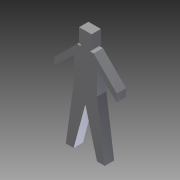
# Autodesk Inventor part: Human_5ft_9in
Saved by Autodesk Inventor 2012 (Build 160160000, 160)
## iProperties
Created: 2013-07-14
Part Number: Human_5ft_9in
Material: Default
Document SubType Name: Modeling
Designer: joe_000
Surface Area: 25016.7 cm^2
Volume: 103629 cm^3
Author: joe_000
Autodesk Inventor part; units mm, degrees
ref_plane "YZ Plane" through (0, 0, 0) normal (1, 0, 0) x (0, 1, 0)
ref_plane "XZ Plane" through (0, 0, 0) normal (0, 1, 0) x (-1, 0, 0)
ref_plane "XY Plane" through (0, 0, 0) normal (0, 0, 1) x (1, 0, 0)
sketch "Sketch1" plane through (0, 0, 0) normal (0, 0, 1) x (1, 0, 0)
  line L0 (101.6, 1752.6) -> (-101.6, 1752.6)
  line L1 (-101.6, 1752.6) -> (-101.6, 1524)
  line L2 (-101.6, 1524) -> (-76.2, 1524)
  line L3 (-135.2884, 1498.6) -> (-513.0009, 1120.8875)
  line L4 (-513.0009, 1120.8875) -> (-513.0009, 995.1639)
  line L5 (-513.0009, 995.1639) -> (-190.5, 1317.6648)
  line L6 (-190.5, 1317.6648) -> (-190.5, 914.4)
  line L7 (190.5, 914.4) -> (190.5, 1317.6648)
  line L8 (190.5, 1317.6648) -> (513.0009, 995.1639)
  line L9 (513.0009, 995.1639) -> (513.0009, 1120.8875)
  line L10 (513.0009, 1120.8875) -> (135.2884, 1498.6)
  line L11 (76.2, 1524) -> (101.6, 1524)
  line L12 (101.6, 1524) -> (101.6, 1752.6)
  line L13 (0, 0) -> (0, 1532.4177)
  line L14 (-135.2884, 1498.6) -> (-76.2, 1498.6)
  line L15 (-76.2, 1498.6) -> (-76.2, 1524)
  line L16 (135.2884, 1498.6) -> (76.2, 1498.6)
  line L17 (76.2, 1498.6) -> (76.2, 1524)
  line L18 (0, 0) -> (-46.4986, 0)
  line L19 (-190.5, 914.4) -> (-190.5, 1317.6648)
  line L20 (-513.0009, 995.1639) -> (-513.0009, 1120.8875)
  line L21 (-135.2884, 1498.6) -> (-76.2, 1498.6)
  line L22 (-76.2, 1524) -> (-101.6, 1524)
  line L23 (-101.6, 1752.6) -> (101.6, 1752.6)
  line L24 (101.6, 1524) -> (76.2, 1524)
  line L25 (76.2, 1498.6) -> (135.2884, 1498.6)
  line L26 (513.0009, 1120.8875) -> (513.0009, 995.1639)
  line L27 (190.5, 1317.6648) -> (190.5, 914.4)
  line L28 (-190.5, 914.4) -> (-317.5, 0)
  line L29 (-317.5, 0) -> (-190.5, 0)
  line L30 (-190.5, 0) -> (0, 711.2)
  line L31 (0, 711.2) -> (190.5, 0)
  line L32 (190.5, 0) -> (317.5, 0)
  line L33 (317.5, 0) -> (190.5, 914.4)
  dimension "d2" = 381
  dimension "d19" = 88.9
  dimension "d23" = 1498.6
  dimension "d24" = 228.6
  dimension "d25" = 203.2
  dimension "d26" = 152.4
  dimension "d27" = 914.4
  dimension "d28" = 711.2
  dimension "d29" = 381
  dimension "d30" = 127
  constraints: 68 end point, 11 parallel, 10 perpendicular, 6 collinear, 6 symmetric about line, 1 point on line, 1 vertical, 8 other
  measures "d2" distance of L6.end L7.start
  measures "d19" distance between parallel lines of L10 L8
  measures "d23" distance between parallel lines of L16 L18
  measures "d24" distance of L11.end L0.start
  measures "d25" distance between parallel lines of L12 L1
  measures "d26" distance between parallel lines of L17 L15
  measures "d27" distance from line of L18 L6.end
  measures "d28" distance from line of L18 L30.end
  measures "d29" distance of L31.end L29.end
  measures "d30" distance of L32.end L31.end
extrude "Extrusion1" add sketch "Sketch1" along normal blind 152.4
body "Solid1"
